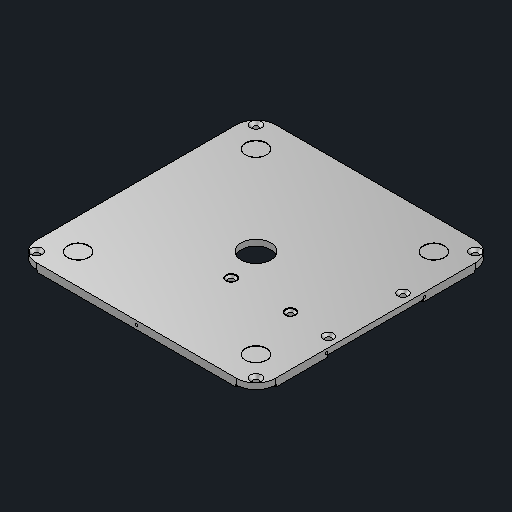
# Autodesk Inventor part: M274_AA_0101_10_Grundplatte
Saved by Autodesk Inventor 2025 (Build 290162010, 162A)
## iProperties
Created: 2024-06-12
Part Number: M274_AA_0101_10_Grundplatte
Material: Aluminium 6061
Document SubType Name: Modeling
Designer: JW4
Density: 2.7 g/cm^3
Appearance: Eloxiert - Hellgrau
Mass: 3172.72 g
Surface Area: 2553.16 cm^2
Volume: 1175.08 cm^3
Author: JW4
Autodesk Inventor part; units mm, degrees
ref_plane "YZ Plane" through (0, 0, 0) normal (1, 0, 0) x (0, 1, 0)
ref_plane "XZ Plane" through (0, 0, 0) normal (0, 1, 0) x (-1, 0, 0)
ref_plane "XY Plane" through (0, 0, 0) normal (0, 0, 1) x (1, 0, 0)
sketch "Skizze1" plane through (0, 0, 0) normal (0, 1, 0) x (-1, 0, 0)
  line L0 (-121, -121) -> (121, -121)
  line L1 (121, -121) -> (121, 121)
  line L2 (121, 121) -> (-121, 121)
  line L3 (-121, 121) -> (-121, -121)
  line L4 (-121, -121) -> (121, 121) construction
  line L5 (121, -121) -> (-121, 121) construction
  point P0 (0, 0)
  dimension "d0" = 242
  dimension "d1" = 242
  constraints: 12 end point, 2 midpoint, 2 parallel, 1 horizontal, 1 perpendicular
  measures "d0" distance of L1.end L2.end
  measures "d1" distance of L0.end L1.end
extrude "Extrusion1" add sketch "Skizze1" along normal blind 8
fillet "Rundung1" radius 20 4 edges at (121, 4, 121) (121, 4, -121) (-121, 4, -121) (-121, 4, 121)
sketch "Skizze6" plane through (0, 8, 0) normal (0, 1, 0) x (1, 0, 0)
  arc A0 (-121, -101) -> (-101, -121) centre (-101, -101) ccw projected
  line L0 (-101, -121) -> (101, -121) projected
  arc A1 (101, -121) -> (121, -101) centre (101, -101) ccw projected
  line L1 (121, -101) -> (121, 101) projected
  arc A2 (121, 101) -> (101, 121) centre (101, 101) ccw projected
  line L2 (101, 121) -> (-101, 121) projected
  arc A3 (-101, 121) -> (-121, 101) centre (-101, 101) ccw projected
  line L3 (-121, 101) -> (-121, -101) projected
  circle A4 centre (0, 0) radius 15
  dimension "d35" = 30
  constraints: 1 centre point, 1 coincident
  measures "d35" diameter of A4
extrude "Extrusion4" cut sketch "Skizze6" against normal blind 10 contours A4
sketch "Skizze9" plane through (0, 8, 0) normal (0, 1, 0) x (1, 0, 0)
  circle A0 centre (0, 0) radius 15 projected
  arc A1 (-121, -101) -> (-101, -121) centre (-101, -101) ccw projected
  line L0 (-101, -121) -> (101, -121) projected
  arc A2 (101, -121) -> (121, -101) centre (101, -101) ccw projected
  line L1 (121, -101) -> (121, 101) projected
  arc A3 (121, 101) -> (101, 121) centre (101, 101) ccw projected
  line L2 (101, 121) -> (-101, 121) projected
  arc A4 (-101, 121) -> (-121, 101) centre (-101, 101) ccw projected
  line L3 (-121, 101) -> (-121, -101) projected
  line L4 (-121, -121) -> (-101, -121)
  line L5 (-101, -121) -> (-101, -101)
  line L6 (-101, -101) -> (-121, -101)
  line L7 (-121, -101) -> (-121, -121)
  line L8 (-121, -121) -> (-101, -101) construction
  line L9 (-101, -121) -> (-121, -101) construction
  line L10 (111, 111) -> (-111, 111)
  line L11 (-111, 111) -> (-111, -111)
  line L12 (-111, -111) -> (111, -111)
  line L13 (111, -111) -> (111, 111)
  line L14 (111, 111) -> (-111, -111) construction
  line L15 (-111, 111) -> (111, -111) construction
  dimension "d69" = 20
  dimension "d70" = 20
  constraints: 24 end point, 6 coincident, 4 midpoint, 4 parallel, 2 horizontal, 2 perpendicular
  measures "d69" distance of L5.end L6.end
  measures "d70" distance of L4.end L5.end
hole "Bohrung3" at (-111, 8, 111) at (-111, 8, -111) at (111, 8, 111) at (111, 8, -111) direction (0, -1, 0) diameter 5.5 depth 20 tip angle 118 countersink diameter 11 countersink angle 90 clearance for "Flachkopfsenkschraube ISO 2009/7046" size "M5" standard "ISO"
sketch "Skizze13" plane through (121, 0, 101) normal (1, 0, 0) x (0, 0, -1)
  line L0 (202, 8) -> (202, 0) projected
  line L1 (0, 8) -> (202, 8) projected
  line L2 (0, 0) -> (0, 8) projected
  line L3 (0, 0) -> (202, 0) projected
  line L4 (0, 0) -> (202, 0) projected
  line L5 (101, 0) -> (101, 8)
  point P0 (101, 0)
  point P1 (51.5, 4)
  point P2 (150.5, 4)
  dimension "d106" = 4
  dimension "d135" = 99
  constraints: 3 midpoint, 2 end point, 1 horizontal alignment, 1 symmetric about line
  measures "d106" distance from line of L3 point (51.5, 4)
  measures "d135" distance of point (150.5, 4) point (51.5, 4)
hole "Bohrung5" at (121, 4, 49.5) at (121, 4, -49.5) direction (-1, 0, 0) diameter 2.459 depth 10 tip angle 118 thread size "M3x0.5" class "6H" standard "ISO Metric profile"
sketch "Skizze14" plane through (-101, 0, 121) normal (0, 0, 1) x (1, 0, 0)
  line L0 (0, 0) -> (0, 8) projected
  line L1 (0, 0) -> (202, 0) projected
  line L2 (202, 8) -> (202, 0) projected
  line L3 (0, 8) -> (202, 8) projected
  point P0 (101, 0)
  point P1 (101, 4)
  point P2 (101, 0)
  dimension "d115" = 4
  constraints: 1 midpoint, 1 vertical alignment
  measures "d115" distance from line of L1 point (101, 4)
hole "Bohrung6" at (0, 4, 121) direction (0, 0, -1) diameter 2.459 depth 10 tip angle 118 thread size "M3x0.5" class "6H" standard "ISO Metric profile"
mirror "Spiegeln2" about plane through (0, 0, 0) normal (1, 0, 0) of "Bohrung5"
mirror "Spiegeln3" about plane through (0, 0, 0) normal (0, 0, 1) of "Bohrung6"
sketch "Skizze15" plane through (0, 0, 0) normal (0, -1, 0) x (1, 0, 0)
  circle A0 centre (111, -111) radius 2.75 projected
  circle A1 centre (111, 111) radius 2.75 projected
  circle A2 centre (-111, -111) radius 2.75 projected
  circle A3 centre (-111, 111) radius 2.75 projected
  circle A4 centre (0, 0) radius 15 projected
  arc A5 (-101, 121) -> (-121, 101) centre (-101, 101) ccw projected
  line L0 (-121, -101) -> (-121, 101) projected
  arc A6 (-121, -101) -> (-101, -121) centre (-101, -101) ccw projected
  line L1 (101, -121) -> (-101, -121) projected
  arc A7 (101, -121) -> (121, -101) centre (101, -101) ccw projected
  line L2 (121, 101) -> (121, -101) projected
  arc A8 (121, 101) -> (101, 121) centre (101, 101) ccw projected
  line L3 (-101, 121) -> (101, 121) projected
  line L4 (-121, 101) -> (-101, 101)
  line L5 (-101, 101) -> (-101, 121)
  line L6 (-101, 121) -> (-121, 121)
  line L7 (-121, 121) -> (-121, 101)
  line L8 (-121, 101) -> (-101, 121) construction
  line L9 (-101, 101) -> (-121, 121) construction
  line L10 (101, 121) -> (121, 121)
  line L11 (121, 121) -> (121, 101)
  line L12 (121, 101) -> (101, 101)
  line L13 (101, 101) -> (101, 121)
  line L14 (101, 121) -> (121, 101) construction
  line L15 (121, 121) -> (101, 101) construction
  line L16 (-121, -121) -> (-101, -121)
  line L17 (-101, -121) -> (-101, -101)
  line L18 (-101, -101) -> (-121, -101)
  line L19 (-121, -101) -> (-121, -121)
  line L20 (-121, -121) -> (-101, -101) construction
  line L21 (-101, -121) -> (-121, -101) construction
  line L22 (101, -121) -> (121, -121)
  line L23 (121, -121) -> (121, -101)
  line L24 (121, -101) -> (101, -101)
  line L25 (101, -101) -> (101, -121)
  line L26 (101, -121) -> (121, -101) construction
  line L27 (121, -121) -> (101, -101) construction
  dimension "d123" = 20
  dimension "d124" = 20
  dimension "d125" = 20
  dimension "d126" = 20
  dimension "d127" = 20
  dimension "d128" = 20
  dimension "d129" = 20
  dimension "d130" = 20
  constraints: 48 end point, 8 midpoint, 8 parallel, 4 horizontal, 4 perpendicular
  measures "d123" distance of L4.end L5.end
  measures "d124" distance of L4.start L4.end
  measures "d125" distance of L11.end L12.end
  measures "d126" distance of L12.end L10.start
  measures "d127" distance of L18.end L17.end
  measures "d128" distance of L16.end L17.end
  measures "d129" distance of L23.end L24.end
  measures "d130" distance of L24.end L22.start
extrude "Extrusion8" cut sketch "Skizze15" against normal blind 2 contours L5 L4 A5 | A8 L12 L13 | L18 L17 A6 | A7 L25 L24
fillet "Rundung6" radius 2 4 edges at (101, 1, 101) (101, 1, -101) (-101, 1, -101) (-101, 1, 101)
fillet "Rundung7" radius 1 8 edges at (101, 1, 121) (121, 1, 101) (121, 1, -101) (101, 1, -121) (-121, 1, -101) (-101, 1, -121) (-121, 1, 101) (-101, 1, 121)
sketch "Skizze17" plane through (0, 0, 0) normal (0, -1, 0) x (1, 0, 0)
  line L0 (141, -47.75) -> (101, -47.75)
  line L1 (101, -47.75) -> (101, 47.75)
  line L2 (101, 47.75) -> (141, 47.75)
  line L3 (141, 47.75) -> (141, -47.75)
  line L4 (121, 101) -> (121, -101) projected
  line L5 (141, -47.75) -> (101, 47.75) construction
  line L6 (101, -47.75) -> (141, 47.75) construction
  point P0 (0, 0)
  point P1 (121, 0)
  point P2 (121, -47.75)
  point P3 (121, 47.75)
  dimension "d138" = 95.5
  dimension "d139" = 20
  constraints: 12 end point, 3 midpoint, 2 parallel, 1 horizontal, 1 perpendicular
  measures "d138" distance of L0.end L1.end
  measures "d139" distance between parallel lines of L4 L1
extrude "Extrusion10" cut sketch "Skizze17" against normal blind 2 contours L0 L1 L2 L4
fillet "Rundung8" radius 2 2 edges at (101, 1, 47.75) (101, 1, -47.75)
fillet "Rundung9" radius 1 2 edges at (121, 1, -47.75) (121, 1, 47.75)
sketch "Skizze19" plane through (0, 8, 0) normal (0, 1, 0) x (1, 0, 0)
  circle A0 centre (111, 111) radius 5.5 projected
  circle A1 centre (111, -111) radius 5.5 projected
  circle A2 centre (-111, 111) radius 5.5 projected
  circle A3 centre (-111, -111) radius 5.5 projected
  circle A4 centre (0, 0) radius 15 projected
  arc A5 (-121, -101) -> (-101, -121) centre (-101, -101) ccw projected
  line L0 (-101, -121) -> (101, -121) projected
  arc A6 (101, -121) -> (121, -101) centre (101, -101) ccw projected
  line L1 (121, -101) -> (121, 101) projected
  arc A7 (121, 101) -> (101, 121) centre (101, 101) ccw projected
  line L2 (101, 121) -> (-101, 121) projected
  arc A8 (-101, 121) -> (-121, 101) centre (-101, 101) ccw projected
  line L3 (-121, 101) -> (-121, -101) projected
  arc A9 (103, 47.75) -> (101, 45.75) centre (103, 45.75) ccw projected
  line L4 (120, 47.75) -> (103, 47.75) projected
  arc A10 (120, 47.75) -> (121, 48.75) centre (120, 48.75) ccw projected
  line L5 (121, -48.75) -> (121, 48.75) projected
  arc A11 (121, -48.75) -> (120, -47.75) centre (120, -48.75) ccw projected
  line L6 (103, -47.75) -> (120, -47.75) projected
  arc A12 (101, -45.75) -> (103, -47.75) centre (103, -45.75) ccw projected
  line L7 (101, 45.75) -> (101, -45.75) projected
  point P0 (111, 37.75)
  point P1 (111, -37.75)
  dimension "d144" = 10
  dimension "d145" = 10
  dimension "d146" = 10
  dimension "d147" = 10
  measures "d144" distance from line of L7 point (111, 37.75)
  measures "d145" distance from line of L4 point (111, 37.75)
  measures "d146" distance from line of L7 point (111, -37.75)
  measures "d147" distance from line of L6 point (111, -37.75)
hole "Bohrung7" at (111, 8, -37.75) at (111, 8, 37.75) direction (0, -1, 0) diameter 5.5 end through all countersink diameter 10.4 countersink angle 90 clearance for "Flachkopfsenkschraube ISO 2009/7046" size "M5" standard "ISO"
sketch "Skizze20" plane through (0, 0, 0) normal (0, -1, 0) x (1, 0, 0)
  arc A0 (120, 47.75) -> (121, 48.75) centre (120, 48.75) ccw projected
  line L0 (121, 100) -> (121, 48.75) projected
  arc A1 (121, 100) -> (120, 101) centre (120, 100) ccw projected
  line L1 (120, 101) -> (103, 101) projected
  arc A2 (101, 103) -> (103, 101) centre (103, 103) ccw projected
  line L2 (101, 103) -> (101, 120) projected
  arc A3 (101, 120) -> (100, 121) centre (100, 120) ccw projected
  line L3 (-100, 121) -> (100, 121) projected
  arc A4 (-100, 121) -> (-101, 120) centre (-100, 120) ccw projected
  line L4 (-101, 120) -> (-101, 103) projected
  arc A5 (-103, 101) -> (-101, 103) centre (-103, 103) ccw projected
  line L5 (-103, 101) -> (-120, 101) projected
  arc A6 (-120, 101) -> (-121, 100) centre (-120, 100) ccw projected
  line L6 (-121, -100) -> (-121, 100) projected
  arc A7 (-121, -100) -> (-120, -101) centre (-120, -100) ccw projected
  line L7 (-120, -101) -> (-103, -101) projected
  arc A8 (-101, -103) -> (-103, -101) centre (-103, -103) ccw projected
  line L8 (-101, -103) -> (-101, -120) projected
  arc A9 (-101, -120) -> (-100, -121) centre (-100, -120) ccw projected
  line L9 (100, -121) -> (-100, -121) projected
  arc A10 (100, -121) -> (101, -120) centre (100, -120) ccw projected
  line L10 (101, -120) -> (101, -103) projected
  arc A11 (103, -101) -> (101, -103) centre (103, -103) ccw projected
  line L11 (103, -101) -> (120, -101) projected
  arc A12 (120, -101) -> (121, -100) centre (120, -100) ccw projected
  line L12 (121, -48.75) -> (121, -100) projected
  arc A13 (121, -48.75) -> (120, -47.75) centre (120, -48.75) ccw projected
  line L13 (120, -47.75) -> (103, -47.75) projected
  arc A14 (101, -45.75) -> (103, -47.75) centre (103, -45.75) ccw projected
  line L14 (101, -45.75) -> (101, 45.75) projected
  arc A15 (103, 47.75) -> (101, 45.75) centre (103, 45.75) ccw projected
  line L15 (103, 47.75) -> (120, 47.75) projected
  circle A16 centre (0, 0) radius 15 projected
  line L16 (-101, -27.5) -> (101, -27.5)
  line L17 (101, -27.5) -> (101, 27.5)
  line L18 (101, 27.5) -> (-101, 27.5)
  line L19 (-101, 27.5) -> (-101, -27.5)
  line L20 (-101, -27.5) -> (101, 27.5) construction
  line L21 (101, -27.5) -> (-101, 27.5) construction
  line L22 (-25, -27.5) -> (-25, 27.5)
  line L23 (101, -45.75) -> (101, 45.75) projected
  dimension "d155" = 55
  dimension "d156" = 25
  constraints: 14 end point, 3 parallel, 3 point on line, 2 midpoint, 1 horizontal, 1 perpendicular
  measures "d155" distance between parallel lines of L18 L16
  measures "d156" distance from line of L22 point (0, 0)
extrude "Extrusion11" cut sketch "Skizze20" against normal blind 2 contours L14 L16 L22 L18
fillet "Rundung10" radius 1 2 edges at (101, 1, 27.5) (101, 1, -27.5)
fillet "Rundung11" radius 3 2 edges at (-25, 1, -27.5) (-25, 1, 27.5)
sketch "Skizze21" plane through (0, 0, 0) normal (0, -1, 0) x (1, 0, 0)
  arc A0 (101, -28.5) -> (100, -27.5) centre (100, -28.5) ccw projected
  line L0 (100, -27.5) -> (-22, -27.5) projected
  arc A1 (-25, -24.5) -> (-22, -27.5) centre (-22, -24.5) ccw projected
  line L1 (-25, -24.5) -> (-25, 24.5) projected
  arc A2 (-22, 27.5) -> (-25, 24.5) centre (-22, 24.5) ccw projected
  line L2 (-22, 27.5) -> (100, 27.5) projected
  arc A3 (100, 27.5) -> (101, 28.5) centre (100, 28.5) ccw projected
  line L3 (101, 28.5) -> (101, 45.75) projected
  arc A4 (103, 47.75) -> (101, 45.75) centre (103, 45.75) ccw projected
  line L4 (103, 47.75) -> (120, 47.75) projected
  arc A5 (120, 47.75) -> (121, 48.75) centre (120, 48.75) ccw projected
  line L5 (121, 100) -> (121, 48.75) projected
  arc A6 (121, 100) -> (120, 101) centre (120, 100) ccw projected
  line L6 (120, 101) -> (103, 101) projected
  arc A7 (101, 103) -> (103, 101) centre (103, 103) ccw projected
  line L7 (101, 103) -> (101, 120) projected
  arc A8 (101, 120) -> (100, 121) centre (100, 120) ccw projected
  line L8 (-100, 121) -> (100, 121) projected
  arc A9 (-100, 121) -> (-101, 120) centre (-100, 120) ccw projected
  line L9 (-101, 120) -> (-101, 103) projected
  arc A10 (-103, 101) -> (-101, 103) centre (-103, 103) ccw projected
  line L10 (-103, 101) -> (-120, 101) projected
  arc A11 (-120, 101) -> (-121, 100) centre (-120, 100) ccw projected
  line L11 (-121, -100) -> (-121, 100) projected
  arc A12 (-121, -100) -> (-120, -101) centre (-120, -100) ccw projected
  line L12 (-120, -101) -> (-103, -101) projected
  arc A13 (-101, -103) -> (-103, -101) centre (-103, -103) ccw projected
  line L13 (-101, -103) -> (-101, -120) projected
  arc A14 (-101, -120) -> (-100, -121) centre (-100, -120) ccw projected
  line L14 (100, -121) -> (-100, -121) projected
  arc A15 (100, -121) -> (101, -120) centre (100, -120) ccw projected
  line L15 (101, -120) -> (101, -103) projected
  arc A16 (103, -101) -> (101, -103) centre (103, -103) ccw projected
  line L16 (103, -101) -> (120, -101) projected
  arc A17 (120, -101) -> (121, -100) centre (120, -100) ccw projected
  line L17 (121, -48.75) -> (121, -100) projected
  arc A18 (121, -48.75) -> (120, -47.75) centre (120, -48.75) ccw projected
  line L18 (120, -47.75) -> (103, -47.75) projected
  arc A19 (101, -45.75) -> (103, -47.75) centre (103, -45.75) ccw projected
  line L19 (101, -45.75) -> (101, -28.5) projected
  circle A20 centre (70.5, 35.6) radius 5.5
  line L20 (121, 48.75) -> (121, -48.75) projected
  point P0 (0, 0)
  point P1 (121, 0)
  dimension "d161" = 11
  dimension "d162" = 50.5
  dimension "d163" = 35.6
  constraints: 1 centre point, 1 midpoint
  measures "d161" diameter of A20
  measures "d162" distance from line of L20 A20.centre
  measures "d163" vertical distance of A20.centre point (121, 0)
extrude "Extrusion12" cut sketch "Skizze21" against normal blind 2 contours A20
sketch "Skizze22" plane through (0, 8, 0) normal (0, 1, 0) x (1, 0, 0)
  circle A0 centre (111, -37.75) radius 5.2 projected
  circle A1 centre (111, 37.75) radius 5.2 projected
  circle A2 centre (111, 111) radius 5.5 projected
  circle A3 centre (111, -111) radius 5.5 projected
  circle A4 centre (-111, 111) radius 5.5 projected
  circle A5 centre (-111, -111) radius 5.5 projected
  circle A6 centre (0, 0) radius 15 projected
  arc A7 (-121, -101) -> (-101, -121) centre (-101, -101) ccw projected
  line L0 (-101, -121) -> (101, -121) projected
  arc A8 (101, -121) -> (121, -101) centre (101, -101) ccw projected
  line L1 (121, -101) -> (121, 101) projected
  arc A9 (121, 101) -> (101, 121) centre (101, 101) ccw projected
  line L2 (101, 121) -> (-101, 121) projected
  arc A10 (-101, 121) -> (-121, 101) centre (-101, 101) ccw projected
  line L3 (-121, 101) -> (-121, -101) projected
  circle A11 centre (70.5, -35.6) radius 5.5 projected
hole "Bohrung8" at (70.5, 8, 35.6) direction (0, -1, 0) diameter 5.5 depth 8 countersink diameter 10.4 countersink angle 90 clearance for "Flachkopfsenkschraube ISO 2009/7046" size "M5" standard "ISO"
pattern_linear "Rechteckige Anordnung1" count 2 spacing 60 along (-1, 0, 0) of "Bohrung8", "Extrusion12"
sketch "Skizze23" plane through (0, 8, 0) normal (0, 1, 0) x (1, 0, 0)
  circle A0 centre (10.5, -35.6) radius 5.2 projected
  circle A1 centre (70.5, -35.6) radius 5.2 projected
  circle A2 centre (111, -37.75) radius 5.2 projected
  circle A3 centre (111, 37.75) radius 5.2 projected
  circle A4 centre (111, 111) radius 5.5 projected
  circle A5 centre (111, -111) radius 5.5 projected
  circle A6 centre (-111, 111) radius 5.5 projected
  circle A7 centre (-111, -111) radius 5.5 projected
  circle A8 centre (0, 0) radius 15 projected
  arc A9 (-121, -101) -> (-101, -121) centre (-101, -101) ccw projected
  line L0 (-101, -121) -> (101, -121) projected
  arc A10 (101, -121) -> (121, -101) centre (101, -101) ccw projected
  line L1 (121, -101) -> (121, 101) projected
  arc A11 (121, 101) -> (101, 121) centre (101, 101) ccw projected
  line L2 (101, 121) -> (-101, 121) projected
  arc A12 (-101, 121) -> (-121, 101) centre (-101, 101) ccw projected
  line L3 (-121, 101) -> (-121, -101) projected
  line L4 (-90, 90) -> (90, 90)
  line L5 (90, 90) -> (90, -90)
  line L6 (90, -90) -> (-90, -90)
  line L7 (-90, -90) -> (-90, 90)
  line L8 (-90, 90) -> (90, -90) construction
  line L9 (90, 90) -> (-90, -90) construction
  circle A13 centre (90, 90) radius 10.5
  circle A14 centre (90, -90) radius 10.5
  circle A15 centre (-90, -90) radius 10.5
  circle A16 centre (-90, 90) radius 10.5
  dimension "d176" = 180
  dimension "d177" = 180
  dimension "d178" = 21
  dimension "d179" = 21
  dimension "d180" = 21
  dimension "d181" = 21
  constraints: 12 end point, 4 centre point, 4 coincident, 2 midpoint, 2 parallel, 1 horizontal, 1 perpendicular
  measures "d176" distance of L4.end L5.end
  measures "d177" distance of L4.start L4.end
  measures "d178" diameter of A13
  measures "d179" diameter of A14
  measures "d180" diameter of A15
  measures "d181" diameter of A16
extrude "Extrusion13" cut sketch "Skizze23" against normal blind 0.5 contours A0 | A1 | A8 | L7 A16 L4 | L4 A16 L7 | A13 L5 L4 | L4 L5 A13 | A15 L6 L7 | L7 L6 A15 | A14 L6 L5 | L5 L6 A14
